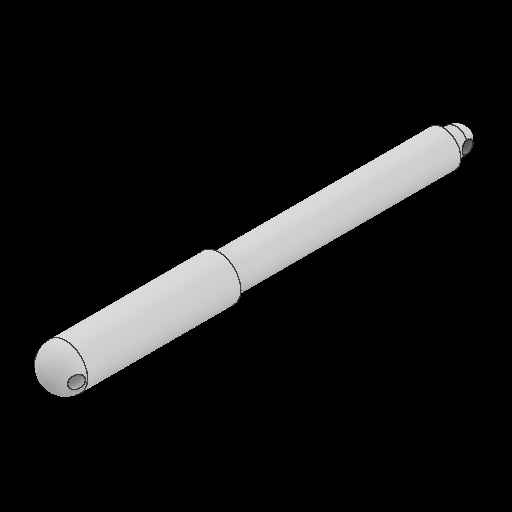
# Autodesk Inventor part: ANT-35
Saved by Autodesk Inventor 2025.2 (Build 292293000, 293)
## iProperties
Created: 2026-01-14
Part Number: ANT-35
Material: Generic
Document SubType Name: Modeling
Designer: valer
Density: 1 g/cm^3
Appearance: Default
Author: valer
Autodesk Inventor part; units mm, degrees
ref_plane "YZ Plane" through (0, 0, 0) normal (1, 0, 0) x (0, 1, 0)
ref_plane "XZ Plane" through (0, 0, 0) normal (0, 1, 0) x (-1, 0, 0)
ref_plane "XY Plane" through (0, 0, 0) normal (0, 0, 1) x (1, 0, 0)
sketch "Sketch1" plane through (0, 0, 0) normal (0, 0, 1) x (1, 0, 0)
  circle A0 centre (0, 0) radius 17.5
  dimension "D" = 35
  constraints: 1 centre point, 1 coincident
  measures "D" diameter of A0
extrude "Extrusion1" add sketch "Sketch1" along normal blind 121.5
sketch "Sketch2" plane through (0, 0, 0) normal (0, 1, 0) x (-1, 0, 0)
  line L0 (17.5, 121.5) -> (-17.5, 121.5) projected
  line L1 (0, 121.5) -> (0, 139)
  arc A0 (0, 139) -> (-17.5, 121.5) centre (0, 121.5) ccw
  line L2 (-17.5, 0) -> (-17.5, 121.5) construction
  point P0 (0, 0)
  dimension "d3" = 17.5
  constraints: 2 end point, 2 point on circle, 1 centre point, 1 midpoint, 1 tangent, 1 vertical
  measures "d3" distance of L1.start L1.end
revolve "Revolution1" add sketch "Sketch2" angle 360 about axis through (0, 0, 121.5) along (0, 0, 1)
sketch "Sketch3" plane through (0, 0, 0) normal (0, 0, -1) x (-1, 0, 0)
  circle A0 centre (0, 0) radius 17.5 projected
  circle A1 centre (0, 0) radius 14
  dimension "d5" = 28
  constraints: 1 centre point, 1 coincident
  measures "d5" diameter of A1
extrude "Extrusion2" add sketch "Sketch3" along normal blind 178 contours A1
sketch "Sketch4" plane through (0, 0, -178) normal (0, 0, -1) x (-1, 0, 0)
  circle A0 centre (0, 0) radius 10
  dimension "d8" = 20
  constraints: 1 centre point, 1 coincident
  measures "d8" diameter of A0
extrude "Extrusion3" add sketch "Sketch4" along normal blind 20
fillet "Fillet1" radius 10 1 edges at (10, 0, -198)
sketch "Sketch5" plane through (0, 0, 0) normal (1, 0, 0) x (0, 1, 0)
  circle A0 centre (0, 128.1186) radius 5
  line L0 (-10, -188) -> (10, -188) projected
  circle A1 centre (0, -188) radius 5
  point P0 (0, 0)
  dimension "d12" = 10
  dimension "d13" = 10
  constraints: 2 centre point, 1 midpoint
  measures "d12" diameter of A0
  measures "d13" diameter of A1
extrude "Extrusion4" cut sketch "Sketch5" along normal through all both and the other way through all
body "Solid1"
